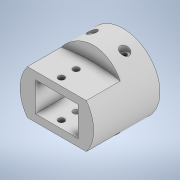
# Autodesk Inventor part: RL_spider_leg_mount
Saved by Autodesk Inventor 2022 (Build 260153000, 153)
## iProperties
Created: 2021-09-28
Part Number: RL_spider_leg_mount
Material: Generic
Document SubType Name: Modeling
Designer: james
Density: 1 g/cm^3
Appearance: Default
Author: james
Autodesk Inventor part; units mm, degrees
ref_plane "YZ Plane" through (0, 0, 0) normal (1, 0, 0) x (0, 1, 0)
ref_plane "XY Plane" through (0, 0, 0) normal (0, 0, 1) x (1, 0, 0)
sketch "Sketch1" plane through (0, 0, 0) normal (0, 0, 1) x (1, 0, 0)
  circle A0 centre (0, 0) radius 25
  line L0 (-14.5, 17.25) -> (14.5, 17.25)
  line L1 (14.5, 17.25) -> (14.5, -17.25)
  line L2 (14.5, -17.25) -> (-14.5, -17.25)
  line L3 (-14.5, -17.25) -> (-14.5, 17.25)
  dimension "d0" = 50
  dimension "d1" = 29
  dimension "d2" = 34.5
  dimension "d3" = 14.5
  dimension "d4" = 17.25
  constraints: 8 end point, 2 parallel, 1 centre point, 1 coincident, 1 horizontal, 1 perpendicular
  measures "d0" diameter of A0
  measures "d1" distance of L0.start L0.end
  measures "d2" distance of L2.end L0.start
  measures "d3" distance from line of point (0, 0) L3
  measures "d4" distance from line of point (0, 0) L0
extrude "Extrusion1" add sketch "Sketch1" along normal blind 30 contours A0 | L0 L1 L2 L3
sketch "Sketch2" plane through (0, 0, 30) normal (0, 0, 1) x (1, 0, 0)
  circle A0 centre (0, 0) radius 25 projected
  line L0 (-20, 15) -> (20, 15)
  line L1 (-20, -15) -> (20, -15)
  dimension "d14" = 30
  dimension "d15" = 15
  constraints: 4 end point, 4 point on circle, 2 horizontal
  measures "d14" distance between parallel lines of L0 L1
  measures "d15" distance from line of L0 A0.centre
extrude "Extrusion2" add sketch "Sketch2" along normal blind 15 contours A0 L1 L0
sketch "Sketch4" plane through (-20, 15, 30) normal (0, 1, 0) x (1, 0, 0)
  circle A0 centre (20, -90) radius 100
  line L0 (40, -15) -> (0, -15) projected
  line L1 (-5, 30) -> (-5, -15) projected
  point P0 (20, 30)
  dimension "d16" = 75
  dimension "d17" = 25
  dimension "d18" = 200
  constraints: 1 centre point
  measures "d16" distance from line of A0.centre L0
  measures "d17" distance from line of A0.centre L1
  measures "d18" diameter of A0
extrude "Extrusion4" cut sketch "Sketch4" along normal blind 10
mirror "Mirror1" about plane through (0, 0, 0) normal (0, 1, 0) of "Extrusion4"
sketch "Sketch5" plane through (0, 0, 0) normal (0, 0, -1) x (-1, 0, 0)
  line L0 (14.5, -17.25) -> (-14.5, -17.25)
  line L1 (-14.5, -17.25) -> (-14.5, 17.25)
  line L2 (-14.5, 17.25) -> (14.5, 17.25)
  line L3 (14.5, 17.25) -> (14.5, -17.25)
  point P0 (0, 0)
  dimension "d21" = 34.5
  dimension "d22" = 29
  dimension "d23" = 17.25
  dimension "d24" = 14.5
  constraints: 8 end point, 2 parallel, 1 horizontal, 1 perpendicular
  measures "d21" distance between parallel lines of L2 L0
  measures "d22" distance of L0.start L0.end
  measures "d23" distance from line of point (0, 0) L0
  measures "d24" distance from line of point (0, 0) L3
extrude "Extrusion5" cut sketch "Sketch5" against normal blind 17
ref_plane "Work Plane1" through (0, 25, 0) normal (0, 1, 0) x (-1, 0, 0)
sketch "Sketch6" plane through (0, 25, 0) normal (0, 1, 0) x (-1, 0, 0)
  circle A0 centre (-11, 10) radius 1.5
  circle A1 centre (11, 10) radius 1.5
  line L0 (25, 0) -> (-25, 0) projected
  line L1 (-14.5, 0) -> (-14.5, 17) projected
  point P0 (0, 0)
  point P1 (-14.5, 16.0568)
  dimension "d28" = 3
  dimension "d29" = 3
  dimension "d30" = 10
  dimension "d31" = 10
  dimension "d32" = 22
  dimension "d33" = 3.5
  constraints: 2 centre point
  measures "d28" diameter of A0
  measures "d29" diameter of A1
  measures "d30" distance from line of L0 A0.centre
  measures "d31" distance from line of L0 A1.centre
  measures "d32" distance of A1.centre A0.centre
  measures "d33" distance from line of A0.centre L1
extrude "Extrusion6" cut sketch "Sketch6" against normal blind 50
sketch "Sketch7" plane through (0, 25, 0) normal (0, 1, 0) x (-1, 0, 0)
  circle A0 centre (-11, 10) radius 1.5 projected
  circle A1 centre (-11, 10) radius 3
  circle A2 centre (11, 10) radius 1.5 projected
  circle A3 centre (11, 10) radius 3
  point P0 (0, 0)
  dimension "d36" = 6
  dimension "d37" = 6
  constraints: 2 centre point, 2 coincident
  measures "d36" diameter of A1
  measures "d37" diameter of A3
extrude "Extrusion7" cut sketch "Sketch7" against normal blind 5 contours A0 | A1 | A2 | A3
mirror "Mirror2" about plane through (0, 0, 0) normal (0, 1, 0) of "Extrusion7"
sketch "Sketch9" plane through (0, 0, 45) normal (0, 0, 1) x (1, 0, 0)
  line L0 (-14.5, 10) -> (14.5, 10)
  line L1 (14.5, 10) -> (14.5, -10)
  line L2 (14.5, -10) -> (-14.5, -10)
  line L3 (-14.5, -10) -> (-14.5, 10)
  line L4 (20, 15) -> (-20, 15) projected
  line L5 (-20, -15) -> (20, -15) projected
  point P0 (0, 0)
  dimension "d57" = 29
  dimension "d58" = 14.5
  dimension "d64" = 5
  dimension "d65" = 5
  constraints: 8 end point, 2 parallel, 1 horizontal, 1 perpendicular
  measures "d57" distance of L0.start L0.end
  measures "d58" distance from line of point (0, 0) L3
  measures "d64" distance between parallel lines of L4 L0
  measures "d65" distance between parallel lines of L5 L2
extrude "Extrusion9" cut sketch "Sketch9" against normal blind 40
chamfer "Chamfer1" distance 7.25 angle 45 2 edges at (0, 10, 17) (0, -10, 17)
sketch "Sketch10" plane through (-20, -15, 45) normal (0, -1, 0) x (1, 0, 0)
  circle A0 centre (18.0952, -5) radius 2.0666
  circle A1 centre (18.0952, -15) radius 2.0679
  line L0 (0, 0) -> (40, 0) projected
  line L1 (7.0094, -25) -> (36.1661, -25)
  arc A2 (0, -22.9796) -> (40, -22.9796) centre (20, 75) ccw projected
  point P0 (20, -45)
  point P1 (18.0952, -25)
  point P2 (32.5952, -28.9432)
  dimension "d66" = 15
  dimension "d67" = 5
  constraints: 2 centre point, 2 end point, 1 horizontal, 1 tangent
  measures "d66" distance from line of L0 A1.centre
  measures "d67" distance from line of L0 A0.centre
extrude "Extrusion10" cut sketch "Sketch10" against normal blind 40
equation "\"d3\" = 0.5 * d1"
equation "\"d4\" = 0.5 * d2"
equation "\"d15\" = 0.5 * d14"
equation "\"d23\" = 0.5 * d21"
equation "\"d24\" = 0.5 * d22"
equation "\"d58\" = 0.5 * d57"
equation "\"d65\" = d64"
body "Solid1"
